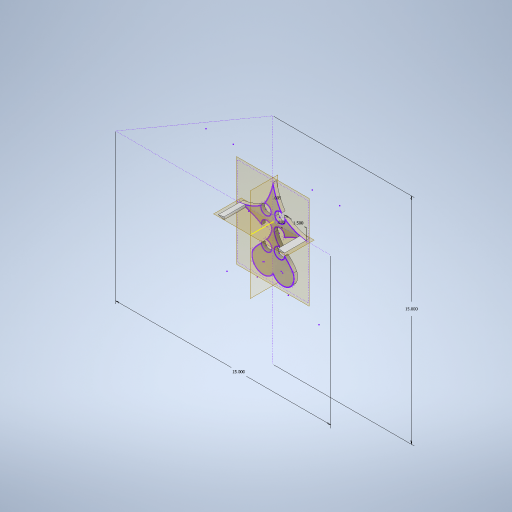
# Autodesk Inventor part: Nobody Emblem Ring
Saved by Autodesk Inventor 2024 (Build 280153000, 153)
## iProperties
Created: 2024-10-02
Part Number: Nobody Emblem Ring
Material: Generic
Document SubType Name: Modeling
Designer: Malik
Density: 1 g/cm^3
Appearance: Default
Author: Malik
Autodesk Inventor part; units mm, degrees
sketch "Sketch1" plane through (0, 0, 0) normal (0, 0, 1) x (1, 0, 0)
  line L0 (-63.346699, 63.7292) -> (61.928792, 63.7292) construction
  line L1 (61.928792, 63.7292) -> (61.928792, -93.080155) construction
  line L2 (61.928792, -93.080155) -> (-63.346699, -93.080155) construction
  line L3 (-63.346699, -93.080155) -> (-63.346699, 63.7292) construction
  line L4 (-0.42552, 162.447522) -> (-0.42552, -218.552478) construction
  line L5 (-278.922376, 0) -> (102.077624, 0) construction
  line L6 (-278.922376, 0) -> (-0.42552, 162.447522) construction
  arc A0 (58.289512, 0.544173) -> (19.231751, -14.479084) centre (81.029762, -116.85958) ccw
  arc A1 (20.189512, 15.840755) -> (58.289512, 0.544173) centre (69.634217, 83.898154) ccw
  arc A2 (3.498748, 10.977204) -> (20.189512, 15.840755) centre (11.994733, 12.892137) ccw
  arc A3 (14.909713, 20.960899) -> (3.498748, 10.977204) centre (11.912504, 12.873603) ccw
  arc A4 (-0.42552, 60.383117) -> (14.909713, 20.960899) centre (117.977264, 83.747962) ccw
  arc A5 (-20.082792, -14.479084) -> (-59.140553, 0.544173) centre (-81.880803, -116.85958) ccw
  arc A6 (-59.140553, 0.544173) -> (-21.040553, 15.840755) centre (-70.485258, 83.898154) ccw
  arc A7 (-21.040553, 15.840755) -> (-4.349789, 10.977204) centre (-12.845774, 12.892137) ccw
  arc A8 (-4.349789, 10.977204) -> (-15.760754, 20.960899) centre (-12.763545, 12.873603) ccw
  arc A9 (-15.760754, 20.960899) -> (-0.42552, 60.383117) centre (-118.828305, 83.747962) ccw
  arc A10 (-3.171758, -14.479084) -> (-20.082792, -14.479084) centre (-11.627275, -12.159576) ccw
  arc A11 (-20.749333, -42.108587) -> (-13.062786, -33.254463) centre (-11.867981, -42.055242) ccw
  arc A12 (-13.062786, -33.254463) -> (-3.171758, -14.479084) centre (-43.362152, -5.299473) ccw
  arc A13 (-35.369694, -79.091841) -> (-0.42552, -80.092171) centre (-17.617152, -69.794979) ccw
  arc A14 (-36.518332, -60.771084) -> (-35.369694, -79.091841) centre (-15.42074, -68.644735) ccw
  arc A15 (-20.749333, -42.108587) -> (-36.518332, -60.771084) centre (27.274466, -98.679918) ccw
  arc A16 (19.231751, -14.479084) -> (2.320717, -14.479084) centre (10.776234, -12.159576) ccw
  arc A17 (12.211745, -33.254463) -> (19.898292, -42.108587) centre (11.01694, -42.055242) ccw
  arc A18 (2.320717, -14.479084) -> (12.211745, -33.254463) centre (42.511111, -5.299473) ccw
  arc A19 (-0.42552, -80.092171) -> (34.518653, -79.091841) centre (16.766111, -69.794979) ccw
  arc A20 (34.518653, -79.091841) -> (35.667291, -60.771084) centre (14.569699, -68.644735) ccw
  arc A21 (35.667291, -60.771084) -> (19.898292, -42.108587) centre (-28.125507, -98.679918) ccw
  arc A22 (14.617916, 21.196775) -> (3.374856, 10.94928) centre (11.912504, 12.873603) ccw
  arc A23 (3.374856, 10.94928) -> (20.435276, 15.506372) centre (11.994733, 12.892137) ccw
  arc A24 (20.435276, 15.506372) -> (57.52626, 0.523283) centre (69.634217, 83.898154) ccw
  arc A25 (57.52626, 0.523283) -> (19.431403, -14.210696) centre (81.029762, -116.85958) ccw
  arc A26 (19.431403, -14.210696) -> (2.197514, -14.510029) centre (10.776234, -12.159576) ccw
  arc A27 (2.197514, -14.510029) -> (11.888162, -33.088957) centre (42.511111, -5.299473) ccw
  arc A28 (11.888162, -33.088957) -> (20.019639, -42.378822) centre (11.01694, -42.055242) ccw
  arc A29 (35.552285, -60.826156) -> (20.019639, -42.378822) centre (-28.125507, -98.679918) ccw
  arc A30 (34.406147, -79.032922) -> (35.552285, -60.826156) centre (14.569699, -68.644735) ccw
  arc A31 (-0.42552, -79.842777) -> (34.406147, -79.032922) centre (16.766111, -69.794979) ccw
  arc A32 (-35.257188, -79.032922) -> (-0.42552, -79.842777) centre (-17.617152, -69.794979) ccw
  arc A33 (-36.403326, -60.826156) -> (-35.257188, -79.032922) centre (-15.42074, -68.644735) ccw
  arc A34 (-20.87068, -42.378822) -> (-36.403326, -60.826156) centre (27.274466, -98.679918) ccw
  arc A35 (-20.87068, -42.378822) -> (-12.739203, -33.088957) centre (-11.867981, -42.055242) ccw
  arc A36 (-12.739203, -33.088957) -> (-3.048555, -14.510029) centre (-43.362152, -5.299473) ccw
  arc A37 (-3.048555, -14.510029) -> (-20.282444, -14.210696) centre (-11.627275, -12.159576) ccw
  arc A38 (-20.282444, -14.210696) -> (-58.377301, 0.523283) centre (-81.880803, -116.85958) ccw
  arc A39 (-58.377301, 0.523283) -> (-21.286317, 15.506372) centre (-70.485258, 83.898154) ccw
  arc A40 (-21.286317, 15.506372) -> (-4.225897, 10.94928) centre (-12.845774, 12.892137) ccw
  arc A41 (-4.225897, 10.94928) -> (-15.468957, 21.196775) centre (-12.763545, 12.873603) ccw
  arc A42 (-15.468957, 21.196775) -> (-0.42552, 59.735749) centre (-118.828305, 83.747962) ccw
  arc A43 (-0.42552, 59.735749) -> (14.617916, 21.196775) centre (117.977264, 83.747962) ccw
  arc A44 (2.631504, 10.781734) -> (21.550603, 13.791702) centre (11.994733, 12.892137) ccw
  arc A45 (13.063953, 22.317492) -> (2.631504, 10.781734) centre (11.912504, 12.873603) ccw
  arc A46 (-0.42552, 56.156547) -> (13.063953, 22.317492) centre (117.977264, 83.747962) ccw
  arc A47 (-13.914994, 22.317492) -> (-0.42552, 56.156547) centre (-118.828305, 83.747962) ccw
  arc A48 (-3.482545, 10.781734) -> (-13.914994, 22.317492) centre (-12.763545, 12.873603) ccw
  arc A49 (-22.401644, 13.791702) -> (-3.482545, 10.781734) centre (-12.845774, 12.892137) ccw
  arc A50 (-54.360773, 0.4299) -> (-22.401644, 13.791702) centre (-70.485258, 83.898154) ccw
  arc A51 (-21.26647, -12.743891) -> (-54.360773, 0.4299) centre (-81.880803, -116.85958) ccw
  arc A52 (-2.309275, -14.695398) -> (-21.26647, -12.743891) centre (-11.627275, -12.159576) ccw
  arc A53 (-11.05737, -32.318413) -> (-2.309275, -14.695398) centre (-43.362152, -5.299473) ccw
  arc A54 (-21.461702, -43.905491) -> (-11.05737, -32.318413) centre (-11.867981, -42.055242) ccw
  arc A55 (-21.461702, -43.905491) -> (-35.713006, -61.156188) centre (27.274466, -98.679918) ccw
  arc A56 (-35.713006, -61.156188) -> (-34.582151, -78.679411) centre (-15.42074, -68.644735) ccw
  arc A57 (-34.582151, -78.679411) -> (-0.42552, -78.232522) centre (-17.617152, -69.794979) ccw
  arc A58 (-0.42552, -78.232522) -> (33.731111, -78.679411) centre (16.766111, -69.794979) ccw
  arc A59 (33.731111, -78.679411) -> (34.861965, -61.156188) centre (14.569699, -68.644735) ccw
  arc A60 (34.861965, -61.156188) -> (20.610662, -43.905491) centre (-28.125507, -98.679918) ccw
  arc A61 (10.206329, -32.318413) -> (20.610662, -43.905491) centre (11.01694, -42.055242) ccw
  arc A62 (1.458234, -14.695398) -> (10.206329, -32.318413) centre (42.511111, -5.299473) ccw
  arc A63 (20.415429, -12.743891) -> (1.458234, -14.695398) centre (10.776234, -12.159576) ccw
  arc A64 (53.509732, 0.4299) -> (20.415429, -12.743891) centre (81.029762, -116.85958) ccw
  arc A65 (21.550603, 13.791702) -> (53.509732, 0.4299) centre (69.634217, 83.898154) ccw
  point P0 (0, 0)
  point P1 (-15.887651, 20.960899)
  point P2 (3.820531, 5.071329)
  dimension "d3" = 381
  dimension "d6" = 381
  dimension "d11" = 38.1
  dimension "d18" = 0.127
  dimension "d19" = 0.762
  constraints: 132 point on circle, 66 centre point, 21 symmetric about line, 6 end point, 2 point on line, 2 tangent, 1 horizontal, 1 vertical, 55 other
  measures "d3" distance of L4.start L4.end
  measures "d6" distance of L5.start L5.end
  measures "d11" horizontal distance of A0.start A1.start
  measures "d18" radial gap between concentric circles of A4 A43
  measures "d19" radial gap between concentric circles of A23 A44
sketch "Sketch1 outline for Extrusion1" plane through (0, 0, 0) normal (0, 0, 1) x (1, 0, 0)
  arc A0 (-20.749333, -42.108587) -> (-36.518332, -60.771084) centre (27.274466, -98.679918) ccw
  arc A1 (-13.062786, -33.254463) -> (-20.749333, -42.108587) centre (-11.867981, -42.055242) cw
  arc A2 (-3.171758, -14.479084) -> (-13.062786, -33.254463) centre (-43.362152, -5.299473) cw
  arc A3 (-20.082792, -14.479084) -> (-3.171758, -14.479084) centre (-11.627275, -12.159576) cw
  arc A4 (-59.140553, 0.544173) -> (-20.082792, -14.479084) centre (-81.880803, -116.85958) cw
  arc A5 (-21.040553, 15.840755) -> (-59.140553, 0.544173) centre (-70.485258, 83.898154) cw
  arc A6 (-4.349789, 10.977204) -> (-21.040553, 15.840755) centre (-12.845774, 12.892137) cw
  arc A7 (-15.760754, 20.960899) -> (-4.349789, 10.977204) centre (-12.763545, 12.873603) cw
  arc A8 (-0.42552, 60.383117) -> (-15.760754, 20.960899) centre (-118.828305, 83.747962) cw
  arc A9 (14.909713, 20.960899) -> (-0.42552, 60.383117) centre (117.977264, 83.747962) cw
  arc A10 (3.498748, 10.977204) -> (14.909713, 20.960899) centre (11.912504, 12.873603) cw
  arc A11 (20.189512, 15.840755) -> (3.498748, 10.977204) centre (11.994733, 12.892137) cw
  arc A12 (58.289512, 0.544173) -> (20.189512, 15.840755) centre (69.634217, 83.898154) cw
  arc A13 (19.231751, -14.479084) -> (58.289512, 0.544173) centre (81.029762, -116.85958) cw
  arc A14 (2.320717, -14.479084) -> (19.231751, -14.479084) centre (10.776234, -12.159576) cw
  arc A15 (12.211745, -33.254463) -> (2.320717, -14.479084) centre (42.511111, -5.299473) cw
  arc A16 (19.898292, -42.108587) -> (12.211745, -33.254463) centre (11.01694, -42.055242) cw
  arc A17 (35.667291, -60.771084) -> (19.898292, -42.108587) centre (-28.125507, -98.679918) ccw
  arc A18 (34.518653, -79.091841) -> (35.667291, -60.771084) centre (14.569699, -68.644735) ccw
  arc A19 (-0.42552, -80.092171) -> (34.518653, -79.091841) centre (16.766111, -69.794979) ccw
  arc A20 (-35.369694, -79.091841) -> (-0.42552, -80.092171) centre (-17.617152, -69.794979) ccw
  arc A21 (-36.518332, -60.771084) -> (-35.369694, -79.091841) centre (-15.42074, -68.644735) ccw
extrude "Extrusion1" add sketch "Sketch1 outline for Extrusion1" against normal blind 6.35
sketch "Sketch2" plane through (0, 0, 0) normal (0, 1, 0) x (-1, 0, 0)
  point P0 (0, 0)
sketch "Sketch3" plane through (0, 0, 0) normal (0, 0, 1) x (1, 0, 0)
  arc A0 (20.189512, 15.840755) -> (58.289512, 0.544173) centre (69.634217, 83.898154) ccw
  arc A1 (58.289512, 0.544173) -> (19.231751, -14.479084) centre (81.029762, -116.85958) ccw
  line L0 (47.821262, 2.652948) -> (47.821262, -1.977224)
  line L1 (47.821262, -1.977224) -> (58.289512, 0.544173)
  line L2 (47.821262, 2.652948) -> (58.289512, 0.544173)
  arc A2 (-0.42552, 60.383117) -> (14.909713, 20.960899) centre (117.977264, 83.747962) ccw construction
  line L3 (-0.42552, 60.383117) -> (-0.42552, -89.381829) construction
  line L4 (-48.672303, 2.652948) -> (-48.672303, -1.977224)
  line L5 (-48.672303, -1.977224) -> (-59.140553, 0.544173)
  line L6 (-48.672303, 2.652948) -> (-59.140553, 0.544173)
  point P0 (0, 0)
  constraints: 14 end point, 3 symmetric about line, 2 point on circle, 2 vertical
extrude "Extrusion2" add sketch "Sketch3" along normal blind 38.1
sketch "Sketch4" plane through (0, 0, 0) normal (1, 0, 0) x (0, 1, 0)
  line L0 (0.544173, 0) -> (0.544173, 38.1)
  point P0 (0, 0)
sketch "Sketch5" plane through (0, 0, 0) normal (0, 1, 0) x (-1, 0, 0)
  point P0 (0, 0)
  point P1 (0, 12.7)
sketch "Sketch6" plane through (0, 0, -6.35) normal (0, 0, -1) x (-1, 0, 0)
  point P0 (0, 0)
body "Solid1"
